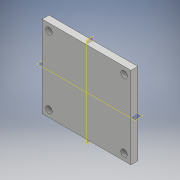
# Autodesk Inventor part: Bottom_part
Saved by Autodesk Inventor 2017 (Build 210142000, 142)
## iProperties
Created: 2020-01-27
Part Number: Bottom_part
Material: Generic
Document SubType Name: Modeling
Designer: Manny
Density: 1 g/cm^3
Appearance: Default
Author: Manny
Autodesk Inventor part; units mm, degrees
ref_plane "YZ Plane" through (0, 0, 0) normal (1, 0, 0) x (0, 1, 0)
ref_plane "XZ Plane" through (0, 0, 0) normal (0, 1, 0) x (-1, 0, 0)
ref_plane "XY Plane" through (0, 0, 0) normal (0, 0, 1) x (1, 0, 0)
sketch "Sketch1" plane through (0, 0, 0) normal (0, 1, 0) x (-1, 0, 0)
  line L0 (0, 0) -> (130, 0)
  line L1 (130, 0) -> (130, -120)
  line L2 (130, -120) -> (0, -120)
  line L3 (0, -120) -> (0, 0)
  dimension "d0" = 120
  dimension "d1" = 130
  constraints: 8 end point, 2 parallel, 1 horizontal, 1 perpendicular
  measures "d0" distance of L0.end L1.end
  measures "d1" distance of L0.start L0.end
extrude "Extrusion1" add sketch "Sketch1" along normal blind 10
sketch "Sketch2" plane through (0, 10, 0) normal (0, 1, 0) x (1, 0, 0)
  circle A0 centre (-120, 110) radius 4.7625
  line L0 (-130, 120) -> (-130, 0) projected
  line L1 (0, 120) -> (-130, 120) projected
  point P0 (0, 0)
  dimension "d4" = 10
  dimension "d5" = 10
  dimension "d6" = 9.525
  constraints: 1 centre point
  measures "d4" distance from line of L0 A0.centre
  measures "d5" distance from line of L1 A0.centre
  measures "d6" diameter of A0
extrude "Extrusion2" cut sketch "Sketch2" against normal blind 10
ref_plane "Work Plane1" through (-65, 0, 0) normal (1, 0, 0) x (0, 0, -1)
ref_plane "Work Plane2" through (0, 0, -60) normal (0, 0, -1) x (-1, 0, 0)
mirror "Mirror1" about plane through (0, 0, -60) normal (0, 0, -1) of "Extrusion2"
mirror "Mirror2" about plane through (-65, 0, 0) normal (1, 0, 0) of "Extrusion2", "Mirror1"
body "Solid1"
